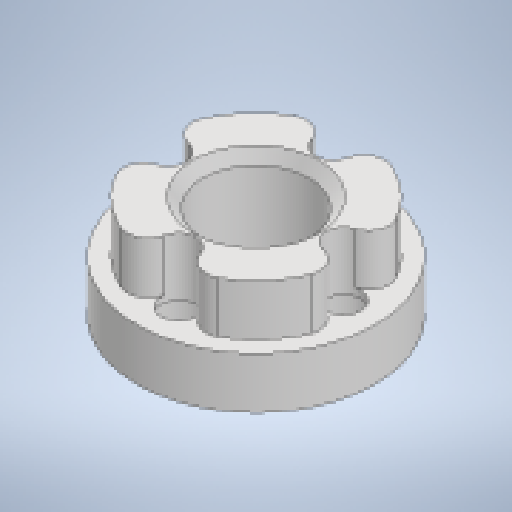
# Autodesk Inventor part: Polea
Saved by Autodesk Inventor 2024 (Build 280153000, 153)
## iProperties
Created: 2025-03-01
Part Number: Polea
Material: Genérico
Document SubType Name: Modeling
Designer: sergi
Density: 1 g/cm^3
Appearance: Valor por defecto
Author: sergi
Autodesk Inventor part; units mm, degrees
ref_plane "YZ Plane" through (0, 0, 0) normal (1, 0, 0) x (0, 1, 0)
ref_plane "XZ Plane" through (0, 0, 0) normal (0, 1, 0) x (-1, 0, 0)
ref_plane "XY Plane" through (0, 0, 0) normal (0, 0, 1) x (1, 0, 0)
sketch "Boceto1" plane through (0, 0, 0) normal (0, 1, 0) x (-1, 0, 0)
  circle A0 centre (0, 0) radius 5.15
  circle A1 centre (0, 0) radius 11.6
  dimension "d0" = 10.3
  dimension "d1" = 23.2
  constraints: 2 centre point, 2 coincident
  measures "d0" diameter of A0
  measures "d1" diameter of A1
extrude "Extrusión1" add sketch "Boceto1" along normal blind 10
sketch "Boceto2" plane through (0, 10, 0) normal (0, 1, 0) x (1, 0, 0)
  circle A0 centre (-0.494, 8.0223) radius 1.425 projected
  circle A1 centre (-0.494, 8.0223) radius 1.425 projected
  circle A2 centre (-8.0223, -0.494) radius 1.425 projected
  circle A3 centre (0.494, -8.0223) radius 1.425 projected
  circle A4 centre (8.0223, 0.494) radius 1.425 projected
  circle A5 centre (0, 0) radius 11 projected
  circle A6 centre (0, 0) radius 1.5 projected
  point P0 (0, 0)
hole "Agujero1" at (-0.494, 10, -8.0223) at (8.0223, 10, -0.494) at (0.494, 10, 8.0223) at (-8.0223, 10, 0.494) direction (0, -1, 0) diameter 3.4 end through all
sketch "Boceto3" plane through (0, 0, 0) normal (0, -1, 0) x (1, 0, 0)
  circle A0 centre (-8.0223, 0.494) radius 1.7 projected
  circle A1 centre (0.494, 8.0223) radius 1.7 projected
  circle A2 centre (8.0223, -0.494) radius 1.7 projected
  circle A3 centre (-0.494, -8.0223) radius 1.7 projected
  circle A4 centre (0, 0) radius 11.6 projected
  circle A5 centre (0, 0) radius 5.15 projected
hole "Agujero2" at (-0.494, 0, -8.0223) at (-8.0223, 0, 0.494) at (0.494, 0, 8.0223) at (8.0223, 0, -0.494) direction (0, 1, 0) diameter 4.5 depth 4 tip angle 118
sketch "Boceto4" plane through (0, 10, 0) normal (0, 1, 0) x (1, 0, 0)
  circle A0 centre (-0.494, 8.0223) radius 1.425 projected
  circle A1 centre (-8.0223, -0.494) radius 1.425 projected
  circle A2 centre (0.494, -8.0223) radius 1.425 projected
  circle A3 centre (8.0223, 0.494) radius 1.425 projected
  circle A4 centre (0, 0) radius 11 projected
  circle A5 centre (0, 0) radius 5 projected
  line L0 (-9.7564, -2.194) -> (-8.0223, -2.194)
  circle A6 centre (-8.0223, -0.494) radius 1.7 projected
  line L1 (-8.0223, 1.206) -> (-9.927, 1.206)
  line L2 (-1.206, -8.0223) -> (-1.206, -9.927)
  line L3 (2.194, -9.7564) -> (2.194, -8.0223)
  line L4 (8.0223, -1.206) -> (9.927, -1.206)
  line L5 (9.7564, 2.194) -> (8.0223, 2.194)
  line L6 (1.206, 8.0223) -> (1.206, 9.927)
  line L7 (-2.194, 9.7564) -> (-2.194, 8.0223)
  arc A7 (-2.194, 9.7564) -> (-9.927, 1.206) centre (0, 0) ccw
  arc A8 (9.7564, 2.194) -> (1.206, 9.927) centre (0, 0) ccw
  arc A9 (-9.7564, -2.194) -> (-1.206, -9.927) centre (0, 0) ccw
  arc A10 (2.194, -9.7564) -> (9.927, -1.206) centre (0, 0) ccw
  circle A11 centre (-0.494, 8.0223) radius 1.425 projected
  circle A12 centre (-8.0223, -0.494) radius 1.425 projected
  circle A13 centre (0.494, -8.0223) radius 1.425 projected
  circle A14 centre (8.0223, 0.494) radius 1.425 projected
  circle A15 centre (0, 0) radius 11 projected
  circle A16 centre (0, 0) radius 1.5 projected
  circle A17 centre (-0.494, 8.0223) radius 1.425 projected
  circle A18 centre (-8.0223, -0.494) radius 1.425 projected
  circle A19 centre (0.494, -8.0223) radius 1.425 projected
  circle A20 centre (8.0223, 0.494) radius 1.425 projected
  circle A21 centre (0, 0) radius 11 projected
  circle A22 centre (0, 0) radius 5 projected
  circle A23 centre (-0.494, 8.0223) radius 1.425 projected
  circle A24 centre (-8.0223, -0.494) radius 1.425 projected
  circle A25 centre (0.494, -8.0223) radius 1.425 projected
  circle A26 centre (8.0223, 0.494) radius 1.425 projected
  circle A27 centre (0, 0) radius 11 projected
  circle A28 centre (0, 0) radius 5 projected
  circle A29 centre (0.494, -8.0223) radius 1.7 projected
  circle A30 centre (8.0223, 0.494) radius 1.7 projected
  circle A31 centre (-0.494, 8.0223) radius 1.7 projected
  circle A32 centre (0, 0) radius 11.6 projected
  dimension "d21" = 360
  constraints: 16 end point, 10 point on circle, 4 centre point, 3 coincident, 2 horizontal, 2 tangent, 25 other
extrude "Extrusión2" cut sketch "Boceto4" against normal blind 5 contours A4 | A32
fillet "Empalme1" radius 2 8 edges at (-9.7564, 7.5, 2.194) (-9.927, 7.5, -1.206) (-2.194, 7.5, -9.7564) (1.206, 7.5, -9.927) (-1.206, 7.5, 9.927) (2.194, 7.5, 9.7564) (9.927, 7.5, 1.206) (9.7564, 7.5, -2.194)
chamfer "Chaflán1" distance 1 angle 45 1 edges at (5.15, 10, 0)
